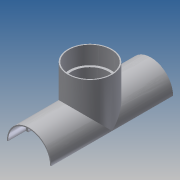
# Autodesk Inventor part: 0T2split
Saved by Autodesk Inventor 2014 SP1 (Build 180222100, 222)
## iProperties
Company: HERA Project
Created: 2013-06-12
Part Number: 0T2split
Material: PVC-Piping
Document SubType Name: Modeling
Designer: David DeBoer
Density: 1.4 g/cm^3
Description: split 2" pvc T
Mass: 405.128 g
Surface Area: 960.349 cm^2
Volume: 289.377 cm^3
Appearance: Smooth - White
Author: David DeBoer
Title: sup
Autodesk Inventor part; units mm, degrees
sketch "Sketch1" plane through (0, 0, 0) normal (0, 0, 1) x (1, 0, 0)
  circle A0 centre (0, 0) radius 31.75
  dimension "d0" = 63.5
  constraints: 1 centre point, 1 coincident
  measures "d0" diameter of A0
extrude "mainBody" add sketch "Sketch1" along normal blind 174.625
sketch "Sketch10" plane through (0, 0, 174.625) normal (0, 0, 1) x (1, 0, 0)
  circle A0 centre (0, 0) radius 30.1625 projected
  circle A1 centre (0, 0) radius 31.75 projected
  point P0 (0, 31.75)
  constraints: 1 vertical alignment, 1 other
ref_plane "Work Plane5" through (0, 31.75, 174.625) normal (0, 1, 0) x (-1, 0, 0)
sketch "Sketch11" plane through (0, 31.75, 174.625) normal (0, 1, 0) x (-1, 0, 0)
  circle A0 centre (0, -87.3125) radius 31.75
  line L0 (31.75, 0) -> (-31.75, 0) projected
  point P0 (0, -174.625)
  dimension "d29" = 87.3125
  dimension "d30" = 63.5
  constraints: 1 centre point
  measures "d29" distance from line of A0.centre L0
  measures "d30" diameter of A0
extrude "TBody" add sketch "Sketch11" along normal blind 38.1 and the other way blind 31.75
sketch "Sketch12" plane through (0, 69.85, 87.3125) normal (0, 1, 0) x (1, 0, 0)
  circle A0 centre (0, 0) radius 31.75 projected
  circle A1 centre (0, 0) radius 30.1625
  point P0 (0, 87.3125)
  dimension "d35" = 60.325
  constraints: 1 centre point, 1 coincident
  measures "d35" diameter of A1
extrude "TSocket" cut sketch "Sketch12" against normal blind 25.4 contours A1
sketch "Sketch13" plane through (0, 44.45, 87.3125) normal (0, 1, 0) x (1, 0, 0)
  circle A0 centre (0, 0) radius 30.1625 projected
  circle A1 centre (0, 0) radius 26.67
  point P0 (0, 87.3125)
  dimension "d39" = 53.34
  constraints: 1 centre point, 1 coincident
  measures "d39" diameter of A1
extrude "TTube" cut sketch "Sketch13" against normal blind 38.1 contours A1
sketch "Sketch14" plane through (0, 0, 174.625) normal (0, 0, 1) x (1, 0, 0)
  circle A0 centre (0, 0) radius 31.75 projected
  circle A1 centre (0, 0) radius 26.67
  dimension "d43" = 53.34
  constraints: 1 centre point, 1 coincident
  measures "d43" diameter of A1
extrude "mainTube" cut sketch "Sketch14" against normal blind 177.8 contours A1
sketch "Sketch15" plane through (0, 0, 174.625) normal (0, 0, 1) x (1, 0, 0)
  circle A0 centre (0, 0) radius 26.67 projected
  circle A1 centre (0, 0) radius 31.75 projected
  circle A2 centre (0, 0) radius 30.1625
  dimension "d47" = 60.325
  constraints: 1 centre point, 1 coincident
  measures "d47" diameter of A2
extrude "mainSocket1" cut sketch "Sketch15" against normal blind 25.4 contours A2
sketch "Sketch16" plane through (0, 0, 0) normal (0, 0, -1) x (-1, 0, 0)
  circle A0 centre (0, 0) radius 26.67 projected
  circle A1 centre (0, 0) radius 31.75 projected
  circle A2 centre (0, 0) radius 30.1625
  dimension "d51" = 60.325
  constraints: 1 centre point, 1 coincident
  measures "d51" diameter of A2
extrude "mainSocket2" cut sketch "Sketch16" against normal blind 25.4 contours A2
sketch "Sketch21" plane through (0, 0, 174.625) normal (0, 0, 1) x (1, 0, 0)
  line L0 (-63.5, -52.3875) -> (63.5, -52.3875)
  line L1 (63.5, -52.3875) -> (63.5, 0)
  line L2 (63.5, 0) -> (-63.5, 0)
  line L3 (-63.5, 0) -> (-63.5, -52.3875)
  constraints: 8 end point, 2 parallel, 1 horizontal, 1 perpendicular
extrude "Extrusion18" cut sketch "Sketch21" against normal blind 203.2
sketch "Sketch23" plane through (-26.67, 0, 25.4) normal (0, -1, 0) x (1, 0, 0)
  line L0 (-3.4925, 149.225) -> (-3.4925, 123.825) projected
  line L1 (-5.08, 149.225) -> (-3.4925, 149.225) projected
  line L2 (-5.08, 61.9125) -> (-5.08, 149.225) projected
  line L3 (-5.08, -25.4) -> (-5.08, 61.9125) projected
  line L4 (-3.4925, -25.4) -> (-5.08, -25.4) projected
  line L5 (-3.4925, 0) -> (-3.4925, -25.4) projected
  line L6 (0, 0) -> (-3.4925, 0) projected
  line L7 (0, 123.825) -> (0, 0) projected
  line L8 (-3.4925, 123.825) -> (0, 123.825) projected
  line L9 (0, 2.288) -> (54.6196, 2.288)
  line L10 (54.6196, 2.288) -> (54.6196, 123.825)
  line L11 (54.6196, 123.825) -> (0, 123.825)
  line L12 (0, 123.825) -> (0, 2.288)
  point P0 (26.67, -25.4)
  constraints: 8 end point, 2 parallel, 1 horizontal, 1 perpendicular, 1 point on line
ref_plane "Work Plane9" through (-26.67, 0, 27.688) normal (0, -0.9665, 0.2565) x (1, 0, 0)
sketch "Sketch24" plane through (-26.67, 0, 27.688) normal (0, -0.9665, 0.2565) x (1, 0, 0)
  circle A0 centre (26.67, 60.0211) radius 30.2
  point P0 (26.67, -26.7614)
  constraints: 1 centre point
extrude "15deg" add sketch "Sketch24" along normal blind 2.54
sketch "Sketch28" plane through (-26.67, -2.455, 28.3397) normal (0, -0.9665, 0.2565) x (1, 0, 0)
  ellipse E0 centre (26.67, 9.5695) end of major axis (26.67, 113.529) minor radius 26.67 (51.8879, 43.4049) -> (51.2161, 50.2241) ccw projected
  ellipse E1 centre (26.67, 61.0148) end of major axis (26.67, 33.4214) minor radius 26.67 (51.2161, 50.2241) -> (46.38, 79.6037) ccw projected
  ellipse E2 centre (26.67, 9.5695) end of major axis (26.67, 113.529) minor radius 26.67 (46.38, 79.6037) -> (45.3561, 83.7461) ccw projected
  arc A0 (45.3561, 83.7461) -> (7.9839, 83.7461) centre (26.67, 60.0211) ccw projected
  ellipse E3 centre (26.67, 9.5695) end of major axis (26.67, 113.529) minor radius 26.67 (7.9839, 83.7461) -> (6.96, 79.6037) ccw projected
  ellipse E4 centre (26.67, 61.0148) end of major axis (26.67, 33.4214) minor radius 26.67 (6.96, 79.6037) -> (2.1239, 50.2241) ccw projected
  ellipse E5 centre (26.67, 9.5695) end of major axis (26.67, 113.529) minor radius 26.67 (2.1239, 50.2241) -> (1.4521, 43.4049) ccw projected
  arc A1 (1.4521, 43.4049) -> (51.8879, 43.4049) centre (26.67, 60.0211) ccw projected
  line L0 (26.67, 90.2212) -> (26.67, 29.8211) construction
  point P0 (26.67, -26.7614)
  constraints: 2 end point, 2 point on circle, 6 other
ref_plane "Work Plane12" through (0, 20.6906, 115.5414) normal (-0.0567, -0.965, 0.2561) x (0, -0.2565, -0.9665)
sketch "Sketch29" plane through (0, 20.6906, 115.5414) normal (-0.0567, -0.965, 0.2561) x (0, -0.2565, -0.9665)
  circle A0 centre (29.8902, 0) radius 6.35
  point P0 (116.9826, -0.5467)
  dimension "d86" = 12.7
  constraints: 1 centre point
  measures "d86" diameter of A0
extrude "Extrusion23" add sketch "Sketch29" along normal mid plane 6.35
sketch "Sketch30" plane through (-0.18, 9.9586, 87.4647) normal (-0.0567, -0.965, 0.2561) x (0.9983, -0.0586, 0)
  circle A0 centre (0, 0) radius 6.35 projected
  point P0 (0.7638, -87.0907)
  point P1 (0, -6.35)
  constraints: 1 vertical alignment, 1 other
ref_plane "Work Plane13" through (-0.2754, 8.335, 81.3265) normal (-0.015, -0.2557, -0.9666) x (0.9983, -0.0586, 0)
sketch "Sketch33" plane through (-0.2754, 8.335, 81.3265) normal (-0.015, -0.2557, -0.9666) x (0.9983, -0.0586, 0)
  circle A0 centre (0.0066, -1.6302) radius 0.7668
  point P0 (0.7638, -12.8026)
  constraints: 1 centre point
extrude "Extrusion24" add sketch "Sketch33" along normal blind 2.54
body "Solid1"
